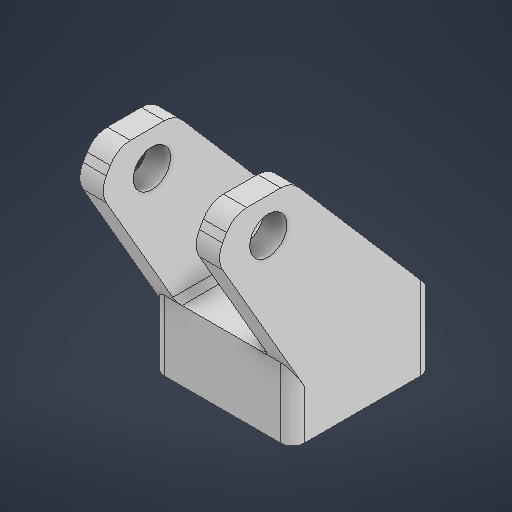
# Autodesk Inventor part: PrzegubDolny
Saved by Autodesk Inventor 2026 (Build 300175000, 175)
## iProperties
Created: 2025-05-01
Part Number: PrzegubDolny
Material: Generic
Document SubType Name: Modeling
Designer: isan
Density: 1 g/cm^3
Appearance: Default
Author: isan
Autodesk Inventor part; units mm, degrees
ref_plane "YZ Plane" through (0, 0, 0) normal (1, 0, 0) x (0, 1, 0)
ref_plane "XZ Plane" through (0, 0, 0) normal (0, 1, 0) x (-1, 0, 0)
ref_plane "XY Plane" through (0, 0, 0) normal (0, 0, 1) x (1, 0, 0)
sketch "Sketch1" plane through (0, 0, 0) normal (0, 0, 1) x (1, 0, 0)
  line L0 (-6, -6) -> (6, -6)
  line L1 (6, -6) -> (6, 6)
  line L2 (6, 6) -> (-6, 6)
  line L3 (-6, 6) -> (-6, -6)
  line L4 (-6, -6) -> (6, 6) construction
  line L5 (6, -6) -> (-6, 6) construction
  point P0 (0, 0)
  dimension "d0" = 12
  dimension "d1" = 12
  constraints: 12 end point, 2 midpoint, 2 parallel, 1 horizontal, 1 perpendicular
  measures "d0" distance of L1.end L2.end
  measures "d1" distance of L0.end L1.end
extrude "Extrusion1" add sketch "Sketch1" along normal blind 6
sketch "Sketch2" plane through (0, 0, 0) normal (0, 0, -1) x (-1, 0, 0)
  circle A0 centre (0, 0) radius 4.1
  dimension "d4" = 8.2
  constraints: 1 centre point, 1 coincident
  measures "d4" diameter of A0
extrude "Extrusion2" cut sketch "Sketch2" against normal blind 4
sketch "Sketch3" plane through (0, 0, 6) normal (0, 0, 1) x (1, 0, 0)
  circle A0 centre (0, 0) radius 1.7
  dimension "d7" = 3.4
  constraints: 1 centre point, 1 coincident
  measures "d7" diameter of A0
extrude "Extrusion3" cut sketch "Sketch3" against normal blind 2
sketch "Sketch5" plane through (6, -6, 0) normal (1, 0, 0) x (0, 0, -1)
  line L0 (0, 12) -> (-6, 12) projected
  line L1 (-6, 0) -> (-6, 12) projected
  line L2 (-6, 12) -> (-6, 0)
  line L3 (-6, 0) -> (-20, -8.0829)
  line L4 (-20, -8.0829) -> (-20, -0.0829)
  line L5 (-20, -0.0829) -> (-6, 12)
  line L6 (0, 0) -> (0, 12) projected
  point P0 (0, 6)
  point P1 (0, 6)
  dimension "d13" = 120
  dimension "d14" = 20
  dimension "d15" = 8
  constraints: 8 end point, 1 collinear, 1 midpoint, 1 parallel
  measures "d13" angle of L1 L3
  measures "d14" horizontal distance of L3.end point (0, 6)
  measures "d15" distance of L3.end L4.end
extrude "Extrusion5" add sketch "Sketch5" against normal blind 2
sketch "Sketch6" plane through (6, -6, 0) normal (1, 0, 0) x (0, 0, -1)
  circle A0 centre (-17, -2.0829) radius 1.6
  line L0 (0, 0) -> (0, 12) projected
  line L1 (-6, 0) -> (-20, -8.0829) projected
  line L2 (-20, -0.0829) -> (-6, 12) projected
  point P0 (0, 6)
  point P1 (0, 6)
  dimension "d18" = 3.2
  dimension "d19" = 17
  dimension "d23" = 2
  constraints: 1 centre point, 1 midpoint
  measures "d18" diameter of A0
  measures "d19" horizontal distance of point (0, 6) A0.centre
  measures "d23" vertical distance of L2.start A0.centre
extrude "Extrusion6" cut sketch "Sketch6" against normal blind 2
mirror "Mirror1" about plane through (0, 0, 0) normal (1, 0, 0) of "Extrusion5", "Extrusion6"
fillet "Fillet1" radius 1 4 edges at (-6, 6, 3) (6, 6, 3) (-6, -6, 3) (6, -6, 3)
fillet "Fillet2" radius 0.5 1 edges at (4.1, 0, 4)
fillet "Fillet3" radius 0.5 2 edges at (-4, 0, 6) (4, 0, 6)
chamfer "Chamfer1" distance 3 angle 45 2 edges at (-5, -14.0829, 20) (5, -14.0829, 20)
fillet "Fillet4" radius 2 6 edges at (-5, -11.0829, 20) (-5, -12.5829, 17.4019) (-5, -6.0829, 20) (5, -6.0829, 20) (5, -11.0829, 20) (5, -12.5829, 17.4019)
body "Solid1"
